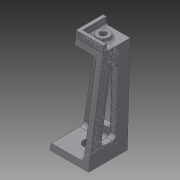
# Autodesk Inventor part: minirambo
Saved by Autodesk Inventor 2014 (Build 180170000, 170)
## iProperties
Created: 2016-05-19
Part Number: minirambo
Material: Generic
Document SubType Name: Modeling
Designer: 101767
Density: 1 g/cm^3
Appearance: Default
Author: 101767
Autodesk Inventor part; units mm, degrees
ref_plane "YZ Plane" through (0, 0, 0) normal (1, 0, 0) x (0, 1, 0)
ref_plane "XZ Plane" through (0, 0, 0) normal (0, 1, 0) x (-1, 0, 0)
sketch "Sketch1" plane through (0, 0, 0) normal (0, 0, 1) x (1, 0, 0)
  line L0 (0, 20) -> (20, 20)
  line L1 (20, 20) -> (20, 0)
  line L2 (20, 0) -> (0, 0)
  line L3 (0, 0) -> (0, 20)
  dimension "d0" = 20
  constraints: 8 end point, 2 parallel, 2 perpendicular, 1 coincident, 1 horizontal
  measures "d0" distance of L0.start L0.end
ref_plane "Work Plane1" through (0, 0, 50) normal (0, 0, 1) x (1, 0, 0)
sketch "Sketch2" plane through (0, 0, 50) normal (0, 0, 1) x (1, 0, 0)
  line L0 (20.75, 20.75) -> (6.75, 20.75)
  line L1 (6.75, 20.75) -> (6.75, 6.75)
  line L2 (6.75, 6.75) -> (20.75, 6.75)
  line L3 (20.75, 6.75) -> (20.75, 20.75)
  line L4 (13.75, 20.75) -> (13.75, 6.75) construction
  line L5 (6.75, 13.75) -> (20.75, 13.75) construction
  line L6 (0, 0) -> (0, 20) construction
  line L7 (20, 0) -> (0, 0) construction
  line L8 (10, 0) -> (10, 32.6821) construction
  line L9 (0, 10) -> (31.2025, 10) construction
  dimension "d4" = 14
  dimension "d13" = 3.75
  dimension "d14" = 3.75
  constraints: 16 end point, 6 midpoint, 4 perpendicular, 2 parallel, 1 horizontal
  measures "d4" distance of L0.start L0.end
  measures "d13" distance between parallel lines of L5 L9
  measures "d14" distance between parallel lines of L8 L4
loft "Loft2" add profiles "Sketch1", "Sketch2"
shell "Shell1" thickness 3 removed faces 2 at (10.625, 1.125, 8.3333) at (1.125, 10.625, 8.3333)
sketch "Sketch3" plane through (6.75, 20.75, 50) normal (0, 0, 1) x (1, 0, 0)
  line L0 (0, 0) -> (14, 0) construction
  line L1 (0, -14) -> (0, 0) construction
  line L2 (14, -14) -> (0, -14) construction
  line L3 (14, 0) -> (14, -14) construction
  line L4 (14, -12.25) -> (1.75, -12.25)
  line L5 (1.75, -12.25) -> (1.75, 0)
  line L6 (1.75, 0) -> (0, 0)
  line L7 (0, 0) -> (0, -14)
  line L8 (0, -14) -> (14, -14)
  line L9 (14, -14) -> (14, -12.25)
  point P0 (-6.75, -20.75)
  dimension "d20" = 1.75
  constraints: 12 end point, 3 collinear, 2 perpendicular, 2 point on line, 1 parallel, 1 other
  measures "d20" distance between parallel lines of L1 L5
extrude "Extrusion3" add sketch "Sketch3" along normal blind 3.5
sketch "Sketch5" plane through (8.5, 8.5, 50) normal (0, 0, 1) x (1, 0, 0)
  line L0 (-1.75, 12.25) -> (-1.75, -1.75) construction
  line L1 (-1.75, -1.75) -> (12.25, -1.75) construction
  line L2 (12.25, 12.25) -> (12.25, 0) construction
  line L3 (0, 12.25) -> (12.25, 12.25) construction
  circle A0 centre (5.25, 5.25) radius 3.3
  point P0 (-8.5, -8.5)
  dimension "d23" = 6.6
  dimension "d24" = 14
  dimension "d25" = 7
  dimension "d26" = 14
  dimension "d27" = 7
  constraints: 1 centre point
  measures "d23" diameter of A0
  measures "d24" distance of L0.start L0.end
  measures "d25" distance from line of A0.centre L1
  measures "d26" distance of L0.end L1.end
  measures "d27" distance from line of A0.centre L0
extrude "Extrusion4" add sketch "Sketch5" along normal blind 2
sketch "Sketch6" plane through (13.75, 13.75, 52) normal (0, 0, 1) x (1, 0, 0)
  circle A0 centre (0, 0) radius 3.3 construction
  circle A1 centre (0, 0) radius 1.65
  point P0 (-13.75, -13.75)
  dimension "d30" = 3.3
  constraints: 1 centre point, 1 coincident
  measures "d30" diameter of A1
extrude "Extrusion5" cut sketch "Sketch6" against normal up to surface (5 mm away)
sketch "Sketch7" plane through (20, 20, 0) normal (0, 0, -1) x (-1, 0, 0)
  line L0 (0, -20) -> (20, -20) construction
  line L1 (20, -20) -> (20, 0) construction
  line L2 (10, -20) -> (10, 0.3197) construction
  line L3 (20, -10) -> (1.197, -10) construction
  circle A0 centre (10, -10) radius 2.75
  dimension "d33" = 5.5
  constraints: 4 end point, 2 midpoint, 2 point on line, 1 centre point, 1 parallel, 1 perpendicular
  measures "d33" diameter of A0
extrude "Extrusion6" cut sketch "Sketch7" against normal up to surface (3 mm away)
sketch "Sketch9" plane through (0, 0, 0) normal (1, 0, 0) x (0, 1, 0)
  line L0 (17.0447, 3) -> (17.7047, 47) construction
  line L1 (17.7047, 47) -> (6.345, 47) construction
  line L2 (0, 0) -> (6.75, 50) construction
  line L3 (17.0447, 3) -> (0.405, 3) construction
  line L4 (10.7154, 42) -> (14.6293, 42)
  line L5 (14.6293, 42) -> (14.1193, 8)
  line L6 (14.1193, 8) -> (6.1254, 8)
  line L7 (10.7154, 42) -> (6.1254, 8)
  line L8 (20, 0) -> (20.75, 50) construction
  dimension "d36" = 5
  dimension "d38" = 5
  dimension "d39" = 5
  dimension "d42" = 6
  constraints: 10 end point, 5 parallel
  measures "d36" distance between parallel lines of L1 L4
  measures "d38" distance between parallel lines of L3 L6
  measures "d39" distance between parallel lines of L2 L7
  measures "d42" distance between parallel lines of L8 L5
extrude "Extrusion7" cut sketch "Sketch9" along normal through all
sketch "Sketch10" plane through (0, 0, 0) normal (0, 1, 0) x (-1, 0, 0)
  line L0 (-20, 0) -> (-20.75, 50) construction
  line L1 (0, 0) -> (-6.75, 50) construction
  line L2 (-14.6293, 42) -> (-10.7154, 42)
  line L3 (-10.7154, 42) -> (-6.1254, 8)
  line L4 (-6.1254, 8) -> (-14.1193, 8)
  line L5 (-14.1193, 8) -> (-14.6293, 42)
  line L6 (0, 0) -> (-20, 0) construction
  line L7 (-6.345, 47) -> (-17.7047, 47) construction
  line L8 (-0.405, 3) -> (-17.0447, 3) construction
  dimension "d43" = 5
  dimension "d44" = 6
  dimension "d51" = 5
  dimension "d52" = 5
  constraints: 8 end point, 3 parallel
  measures "d43" distance between parallel lines of L1 L3
  measures "d44" distance between parallel lines of L0 L5
  measures "d51" distance between parallel lines of L7 L2
  measures "d52" distance between parallel lines of L8 L4
extrude "Extrusion8" cut sketch "Sketch10" along normal through all
fillet "Fillet1" radius 1 3 edges at (14.625, 8.5, 50) (8.5, 14.625, 50) (10.45, 13.75, 50)
fillet "Fillet2" radius 2 13 edges at (8.7248, 17.0447, 3) (17.0447, 8.7248, 3) (17.3747, 17.3747, 25) (17.7047, 12.0248, 47) (12.0248, 17.7047, 47) (14.6293, 19.1298, 42) (10.7154, 19.1298, 42) (6.1254, 18.6198, 8) (14.1193, 18.6198, 8) (18.6198, 6.1254, 8) (18.6198, 14.1193, 8) (19.1298, 10.7154, 42) (19.1298, 14.6293, 42)
sketch "Sketch11" plane through (15.6744, 6.345, 47) normal (0, 0, -1) x (-1, 0, 0)
  line L0 (0, 9.3294) -> (9.3294, 9.3294) construction
  circle A0 centre (1.9244, 7.405) radius 1.65 construction
  line L1 (4.2719, 9.7524) -> (5.1311, 6.5458)
  line L2 (5.1311, 6.5458) -> (2.7837, 4.1984)
  line L3 (2.7837, 4.1984) -> (-0.423, 5.0576)
  line L4 (-0.423, 5.0576) -> (-1.2822, 8.2642)
  line L5 (-1.2822, 8.2642) -> (1.0652, 10.6116)
  line L6 (1.0652, 10.6116) -> (4.2719, 9.7524)
  point P0 (15.6744, -6.345)
  dimension "d55" = 5.75
  dimension "d60" = 45
  constraints: 12 end point, 1 coincident, 13 other
  measures "d55" distance between parallel lines of L2 L5
  measures "d60" angle of L0 L2
extrude "Extrusion9" cut sketch "Sketch11" against normal blind 1.5 and the other way blind 1.5
equation "\"d25\" = 0.5 * d24"
equation "\"d27\" = 0.5 * d26"
body "Solid2"
